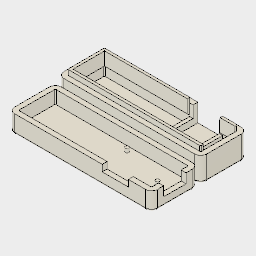
Case for Navilock GPS to Bluetooth v25 (Autodesk Fusion 360 design; units mm, degrees)
Autodesk Fusion 360 part; units mm, degrees
sketch "Circuits sketch" plane through (0, 0, 0) normal (0, 1, 0) x (1, 0, 0)
  line L0 (0.1, 11.325) -> (69.92388, 11.325)
  line L1 (70.02388, 11.225) -> (70.02388, -7.225)
  line L2 (69.92388, -7.325) -> (0.12388, -7.325)
  line L3 (0.02388, -7.225) -> (0.02388, 11.225)
  line L4 (-14.57612, 8) -> (3.42388, 8)
  line L5 (3.42388, 8) -> (3.42388, -4)
  line L6 (3.42388, -4) -> (-14.57612, -4)
  line L7 (-14.57612, -4) -> (-14.57612, 8)
  line L8 (9.22388, 12.325) -> (23.22388, 12.325)
  line L9 (23.22388, 12.325) -> (23.22388, -0.675)
  line L10 (23.22388, -0.675) -> (9.22388, -0.675)
  line L11 (9.22388, -0.675) -> (9.22388, 12.325)
  arc A0 (0.123999, 11.325) -> (0.02388, 11.225) centre (0.12388, 11.225) ccw
  arc A1 (70.02388, 11.225) -> (69.92388, 11.325) centre (69.92388, 11.225) ccw
  arc A2 (69.92388, -7.325) -> (70.02388, -7.225) centre (69.92388, -7.225) ccw
  arc A3 (0.02388, -7.225) -> (0.12388, -7.325) centre (0.12388, -7.225) ccw
  line L12 (-14.57612, 2) -> (70.02388, 2) construction
  arc A4 (73.12388, 11.225) -> (69.92388, 14.425) centre (69.92388, 11.225) ccw
  line L13 (0.12388, 14.425) -> (69.92388, 14.425)
  arc A5 (0.12388, 14.425) -> (-3.07612, 11.225) centre (0.12388, 11.225) ccw
  line L14 (-3.07612, -7.225) -> (-3.07612, 11.225)
  arc A6 (-3.07612, -7.225) -> (0.12388, -10.425) centre (0.12388, -7.225) ccw
  line L15 (69.92388, -10.425) -> (0.12388, -10.425)
  arc A7 (69.92388, -10.425) -> (73.12388, -7.225) centre (69.92388, -7.225) ccw
  line L16 (73.12388, 11.225) -> (73.12388, -7.225)
  arc A8 (70.82388, 11.225) -> (69.92388, 12.125) centre (69.92388, 11.225) ccw
  line L17 (0.12388, 12.125) -> (69.92388, 12.125)
  arc A9 (0.12388, 12.125) -> (-0.77612, 11.225) centre (0.12388, 11.225) ccw
  line L18 (-0.77612, -7.225) -> (-0.77612, 11.225)
  arc A10 (-0.77612, -7.225) -> (0.12388, -8.125) centre (0.12388, -7.225) ccw
  line L19 (69.92388, -8.125) -> (0.12388, -8.125)
  arc A11 (69.92388, -8.125) -> (70.82388, -7.225) centre (69.92388, -7.225) ccw
  line L20 (70.82388, 11.225) -> (70.82388, -7.225)
  circle A12 centre (29.52388, 9.125) radius 1
  circle A13 centre (29.52388, -5.125) radius 1
  circle A14 centre (6.103777, 2) radius 1
  point P0 (0.02388, 2)
  dimension "d17" = 18
  dimension "d18" = 12
  dimension "d19" = 14
  dimension "d20" = 13
  dimension "d32" = 0.1
  dimension "d39" = 5.8
  dimension "d40" = 18.65
  dimension "d41" = 70
  dimension "d43" = 1
  dimension "d76" = 0.8
  dimension "d77" = 2.3
  dimension "d82" = 2
  dimension "d83" = 2
  dimension "d137" = 3.4
  dimension "d139" = 3
  dimension "d140" = 6.079897
  dimension "d151" = 29.5
  measures "d32" radius of A0
  measures "d39" distance of L5 L11
  measures "d40" distance of L0 L2
  measures "d41" distance of L1 L3
  measures "d43" distance of L0 L8
  measures "d76" distance of L0 L17
  measures "d77" distance of L13 L17
  measures "d82" diameter of A12
  measures "d83" diameter of A14
  measures "d137" distance of L3 L5
extrude "Extrude3" add sketch "Circuits sketch" along normal blind 1.6 contours L0 L1 L2 L3 L4 L5 L6 L9 L10 L11 A0 A1 A2 A3 | L0 L9 L10 L11 | L3 L4 L5 L6 | A12 | A13 | A14 picked at (56.775737, 4.276748) picked at (18.557213, 3.325) picked at (1.157213, 4) picked at (30.097841, 9.401405) picked at (29.449706, -4.800024) picked at (6.415186, 1.806801) makes body 1
extrude "Extrude4" add sketch "Circuits sketch" along normal blind 5.1 contours L3 L4 L5 L6 | L3 L4 L6 L18 | L4 L6 L14 L18 | L4 L6 L7 L14 picked at (1.157213, 4) picked at (-0.509454, 4) picked at (-1.542787, 0) picked at (-10.742787, 0) bodies 1
extrude "Extrude5" add sketch "Circuits sketch" along normal blind 14.7 and the other way blind -1.6 contours L0 L9 L11 L17 | L0 L9 L10 L11 | L8 L9 L11 L17 picked at (13.890546, 11.858333) picked at (18.557213, 3.325) picked at (13.890546, 12.258333) bodies 1
move_body "MoveBody7" bodies 1 to x (1, 0, 0) y (0, 1, 0) z (0, 0, 1) at (0, 2, 0)
extrude "Extrude17" add sketch "Circuits sketch" along normal blind 22.49 separate body contours L0 L3 L4 L11 A0 L17 A9 L18 | L0 L1 L2 L3 L4 L5 L6 L9 L10 L11 A0 A1 A2 A3 | L0 L9 L11 L17 | L0 L9 L10 L11 | L0 L1 L2 L3 L6 L9 A1 A2 A3 A8 L17 L18 A10 L19 A11 L20 | L4 L6 L8 L9 L11 A4 L13 A5 L14 A6 L15 A7 L16 A8 L17 A9 L18 A10 L19 A11 L20 | L8 L9 L11 L17 | L3 L4 L5 L6 | L3 L4 L6 L18 | L4 L6 L14 L18 | A12 | A13 | A14 picked at (3.157253, 11.858333) picked at (56.775737, 4.276748) picked at (13.890546, 11.858333) picked at (18.557213, 3.325) picked at (23.390546, -7.858333) picked at (46.657213, -9.658333) picked at (13.890546, 12.258333) picked at (1.157213, 4) picked at (-0.509454, 4) picked at (-1.542787, 0) picked at (30.097841, 9.401405) picked at (29.449706, -4.800024) picked at (6.415186, 1.806801) makes body 2
move_body "MoveBody8" bodies 1 to x (1, 0, 0) y (0, 1, 0) z (0, 0, 1) at (0, 2, 0)
shell "Shell5" thickness 2.6 removed faces 0 bodies 2
move_body "MoveBody9" bodies 1 to x (1, 0, 0) y (0, 1, 0) z (0, 0, 1) at (0, 0.5, 0)
extrude "Extrude18" add sketch "Circuits sketch" along normal blind 4.5 contours A12 | A13 | A14 picked at (30.097841, 9.401405) picked at (29.449706, -4.800024) picked at (6.415186, 1.806801) bodies 2
box "BoxPrimitive2" add length 17.5 width 17.54092 height 4 placed x (0, 0, 1) y (-1, 0, 0) z (0, -1, 0) at (25.04092, 19.89, -14.125) bodies 2
extrude "Extrude19" cut 1 faces at (18.557213, 14.833333, -12.325) along direction (0, 0, -1) mid plane 28 on bodies 1 bodies 2
extrude "Extrude20" cut 1 faces at (-14.57612, 6.2, 0) along direction (1, 0, 0) blind 23 on bodies 1 bodies 2
fillet "Fillet4" radius 1 16 edges at (35.02388, 22.49, 10.425) (72.186621, 22.49, 9.487742) (73.12388, 22.49, -2) (72.186621, 22.49, -13.487742) (35.02388, 22.49, -14.425) (-2.138862, 22.49, -13.487742) (-3.07612, 22.49, -2) (-2.138862, 22.49, 9.487742) (72.186621, 0, -13.487742) (73.12388, 0, -2) (72.186621, 0, 9.487742) (35.02388, 0, 10.425) (-2.138862, 0, 9.487742) (-3.07612, 0, -2) (-2.138862, 0, -13.487742) (35.02388, 0, -14.425) on bodies 2
split "Split3" by plane through (0, 9.6, 0) normal (0, 1, 0) bodies 2 makes body 3 at (23.390546, 22.49, 1.808333)
move_body "MoveBody15" bodies 3 to x (1, 0, 0) y (0, -1, 0) z (0, 0, -1) at (0, 22.4, 22.25)
sketch "Sketch30" plane through (0, 2.51, 0) normal (0, 1, 0) x (-1, 0, 0)
  line L0 (-25.04092, 18.875) -> (-25.04092, 34.075)
  line L1 (-25.04092, 34.075) -> (-69.92388, 34.075)
  arc A0 (-69.92388, 34.075) -> (-70.52388, 33.475) centre (-69.92388, 33.475) ccw
  line L2 (-70.52388, 33.475) -> (-70.52388, 15.025)
  arc A1 (-70.52388, 15.025) -> (-69.92388, 14.425) centre (-69.92388, 15.025) ccw
  line L3 (-69.92388, 14.425) -> (-0.12388, 14.425)
  arc A2 (-0.12388, 14.425) -> (0.47612, 15.025) centre (-0.12388, 15.025) ccw
  line L4 (0.47612, 15.025) -> (0.47612, 33.475)
  arc A3 (0.47612, 33.475) -> (-0.12388, 34.075) centre (-0.12388, 33.475) ccw
  line L5 (-0.12388, 34.075) -> (-7.5, 34.075)
  line L6 (-7.5, 34.075) -> (-7.5, 18.875)
  line L7 (-7.5, 18.875) -> (-25.04092, 18.875)
  line L8 (0.474251, 14.425) -> (-3.525749, 14.425)
  line L9 (-3.61015, 15.83705) -> (0.474251, 15.83705)
  line L10 (0.474251, 15.83705) -> (0.474251, 14.425)
  line L11 (-0.12388, 14.425) -> (-69.92388, 14.425)
  line L12 (-70.525749, 14.425) -> (-33.62388, 14.425)
  line L13 (-37.11015, 15.83705) -> (-33.11015, 15.83705)
  line L14 (-33.025749, 14.425) -> (-37.025749, 14.425)
  line L15 (-3.525749, 34.082) -> (0.474251, 34.082)
  line L16 (0.474251, 34.082) -> (0.474251, 32.708739)
  line L17 (0.474251, 32.708739) -> (-3.490371, 32.708739)
  line L18 (-37.025749, 34.082) -> (-33.025749, 34.082)
  line L19 (-32.990371, 32.708739) -> (-36.990371, 32.708739)
  line L20 (-70.525749, 14.425) -> (-70.521217, 16.242)
  line L21 (-66.525749, 14.425) -> (-70.525749, 14.425)
  line L22 (-70.525749, 34.082) -> (-66.525749, 34.082)
  line L23 (-70.525749, 32.708739) -> (-70.525749, 34.082)
  line L24 (-3.525749, 14.425) -> (-33.025749, 14.425)
  line L25 (-33.11015, 15.83705) -> (-3.61015, 15.83705)
  line L26 (-37.025749, 14.425) -> (-66.525749, 14.425)
  line L27 (-69.117071, 15.83705) -> (-37.11015, 15.83705)
  line L28 (-3.490371, 32.708739) -> (-7.5, 32.708739)
  line L29 (-7.5, 32.708739) -> (-7.5, 34.075)
  line L30 (-7.5, 34.075) -> (-3.525749, 34.075)
  line L31 (-32.990371, 32.708739) -> (-25.04092, 32.708739)
  line L32 (-25.04092, 32.708739) -> (-25.04092, 34.075)
  line L33 (-25.04092, 34.075) -> (-33.025749, 34.075)
  line L34 (-36.990371, 32.708739) -> (-66.580468, 32.708739)
  line L35 (-66.525749, 34.082) -> (-37.025749, 34.082)
  line L36 (-69.117071, 15.83705) -> (-69.117071, 32.708739)
  line L37 (-70.52388, 32.708739) -> (-70.525749, 32.708739)
  line L38 (-70.525749, 32.708739) -> (-70.521217, 16.242)
  line L39 (-66.580468, 32.708739) -> (-69.117071, 32.708739)
  line L40 (-70.52388, 32.708739) -> (-70.525749, 32.708739)
  point P0 (-7.5, 34.075)
  point P1 (-25.04092, 34.075)
extrude "Extrude31" add sketch "Sketch30" along normal blind 13 and the other way blind -5 contours L0 L1 A0 L2 A1 L3 A2 L8 L9 L10 L11 L12 L13 L14 L19 L20 L21 L24 L25 L26 L27 L31 L32 L33 L34 L36 L38 L39 | A3 L5 L6 L16 L17 L28 L29 L30 | L2 L37 L38 L40 picked at (-57.584323, 15.366367) picked at (-1.046667, 33.164159) picked at (-70.524503, 30.44489) bodies 3
chamfer "Chamfer7" distance 1 angle 45 4 edges at (47.078996, 7.51, 32.708739) (69.117071, 7.51, 24.272895) (34.32141, 7.51, 15.83705) (3.512874, 7.51, 32.708739) on bodies 3
hidden bodies 1
equation "d79 = ( 11.245 * 2 ) * 1 mm"
named bodies: "Circuit", "BOTTOM", "TOP"
